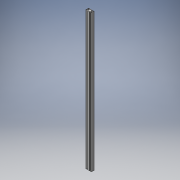
# Autodesk Inventor part: Tslot_2040extrusion_38inch
Saved by Autodesk Inventor 2018 (Build 220112000, 112)
## iProperties
Created: 2020-03-14
Part Number: Tslot_2040extrusion_38inch
Material: Generic
Document SubType Name: Modeling
Designer: natha
Density: 1 g/cm^3
Appearance: Default
Author: natha
Autodesk Inventor part; units mm, degrees
ref_plane "YZ Plane" through (0, 0, 0) normal (1, 0, 0) x (0, 1, 0)
ref_plane "XZ Plane" through (0, 0, 0) normal (0, 1, 0) x (-1, 0, 0)
ref_plane "XY Plane" through (0, 0, 0) normal (0, 0, 1) x (1, 0, 0)
sketch "Sketch1" plane through (0, 0, 0) normal (0, 1, 0) x (-1, 0, 0)
  circle A0 centre (29.9915, -10) radius 2.75
  circle A1 centre (9.9915, -10) radius 2.75
  line L0 (0, 0) -> (0, -6.5)
  line L1 (-0.0085, -20) -> (-0.0085, -13.5)
  line L2 (0, -6.5) -> (0.5, -6.5)
  line L3 (0.5, -6.5) -> (0.5, -7)
  line L4 (0.5, -7) -> (1, -7)
  line L5 (-0.0085, -13.5) -> (0.4915, -13.5)
  line L6 (0.4915, -13.5) -> (0.4915, -13)
  line L7 (0.4915, -13) -> (0.9915, -13)
  line L8 (1, -4.05) -> (3, -4.05)
  line L9 (0.9915, -15.95) -> (2.9915, -15.95)
  line L10 (5.5, -6.5) -> (5.5, -13.5)
  line L11 (5.5, -13.5) -> (2.9915, -15.95)
  line L12 (5.5, -6.5) -> (3, -4.05)
  line L13 (1, -4.05) -> (1, -7)
  line L14 (0.9915, -13) -> (0.9915, -15.95)
  line L15 (-0.0085, -20) -> (6.4915, -20)
  line L16 (6.4915, -20) -> (6.4915, -19.5)
  line L17 (6.4915, -19.5) -> (6.9915, -19.5)
  line L18 (6.9915, -19.5) -> (6.9915, -19)
  line L19 (6.9915, -19) -> (4.0415, -19)
  line L20 (4.0415, -19) -> (4.0415, -17)
  line L21 (13.4915, -20) -> (13.4915, -19.5)
  line L22 (13.4915, -19.5) -> (12.9915, -19.5)
  line L23 (12.9915, -19.5) -> (12.9915, -19)
  line L24 (12.9915, -19) -> (15.9415, -19)
  line L25 (15.9415, -19) -> (15.9415, -17)
  line L26 (15.9415, -17) -> (13.4915, -14.5)
  line L27 (6.4915, -14.5) -> (13.4915, -14.5)
  line L28 (4.0415, -17) -> (6.4915, -14.5)
  line L29 (39.9915, 0) -> (39.9915, -6.5)
  line L30 (39.9915, -6.5) -> (39.4915, -6.5)
  line L31 (39.4915, -6.5) -> (39.4915, -7)
  line L32 (39.4915, -7) -> (38.9915, -7)
  line L33 (38.9915, -7) -> (38.9915, -4.05)
  line L34 (38.9915, -4.05) -> (36.9915, -4.05)
  line L35 (39.9915, -20) -> (39.9915, -13.5)
  line L36 (39.9915, -13.5) -> (39.4915, -13.5)
  line L37 (39.4915, -13.5) -> (39.4915, -13)
  line L38 (39.4915, -13) -> (38.9915, -13)
  line L39 (38.9915, -13) -> (38.9915, -15.95)
  line L40 (38.9915, -15.95) -> (36.9915, -15.95)
  line L41 (34.4915, -6.601) -> (34.4915, -13.5)
  line L42 (34.4915, -13.5) -> (36.9915, -15.95)
  line L43 (34.4915, -6.601) -> (36.9915, -4.05)
  line L44 (39.9915, -20) -> (33.4915, -20)
  line L45 (33.4915, -20) -> (33.4915, -19.5)
  line L46 (33.4915, -19.5) -> (32.9915, -19.5)
  line L47 (32.9915, -19.5) -> (32.9915, -19)
  line L48 (32.9915, -19) -> (35.9415, -19)
  line L49 (35.9415, -19) -> (35.9415, -17)
  line L50 (26.4915, -20) -> (26.4915, -19.5)
  line L51 (26.4915, -19.5) -> (26.9915, -19.5)
  line L52 (26.9915, -19.5) -> (26.9915, -19)
  line L53 (26.9915, -19) -> (24.0415, -19)
  line L54 (24.0415, -19) -> (24.0415, -17)
  line L55 (33.4915, -14.5) -> (26.4915, -14.5)
  line L56 (24.0415, -17) -> (26.4915, -14.5)
  line L57 (33.4915, -14.5) -> (35.9415, -17)
  line L58 (26.4915, -20) -> (13.4915, -20)
  line L59 (39.9915, 0) -> (33.4915, 0)
  line L60 (33.4915, 0) -> (33.4915, -0.5)
  line L61 (33.4915, -0.5) -> (32.9915, -0.5)
  line L62 (32.9915, -0.5) -> (32.9915, -1)
  line L63 (32.9915, -1) -> (35.9415, -1)
  line L64 (35.9415, -1) -> (35.9415, -3)
  line L65 (26.4915, 0) -> (26.4915, -0.5)
  line L66 (26.4915, -0.5) -> (26.9915, -0.5)
  line L67 (26.9915, -0.5) -> (26.9915, -1)
  line L68 (26.9915, -1) -> (24.0415, -1)
  line L69 (24.0415, -1) -> (24.0415, -3)
  line L70 (33.4915, -5.5) -> (26.4915, -5.5)
  line L71 (24.0415, -3) -> (26.4915, -5.5)
  line L72 (35.9415, -3) -> (33.4915, -5.5)
  line L73 (0, 0) -> (6.5, 0)
  line L74 (6.5, 0) -> (6.5, -0.5)
  line L75 (6.5, -0.5) -> (7, -0.5)
  line L76 (7, -0.5) -> (7, -1)
  line L77 (7, -1) -> (4.05, -1)
  line L78 (4.05, -1) -> (4.05, -3)
  line L79 (13.5, 0) -> (13.5, -0.5)
  line L80 (13.5, -0.5) -> (13, -0.5)
  line L81 (13, -0.5) -> (13, -1)
  line L82 (13, -1) -> (15.95, -1)
  line L83 (15.95, -1) -> (15.95, -3)
  line L84 (13.5, -5.5) -> (6.5, -5.5)
  line L85 (6.5, -5.5) -> (4.05, -3)
  line L86 (15.95, -3) -> (13.5, -5.5)
  line L87 (13.5, 0) -> (26.4915, 0)
  dimension "d0" = 40
  dimension "d1" = 20
  dimension "d2" = 5.5
  dimension "d3" = 5.5
  dimension "d4" = 20
  dimension "d11" = 6.5
  dimension "d12" = 6.5
  dimension "d13" = 0.5
  dimension "d14" = 0.5
  dimension "d15" = 0.5
  dimension "d16" = 0.5
  dimension "d17" = 0.5
  dimension "d18" = 0.5
  dimension "d19" = 5.5
  dimension "d20" = 11.9
  dimension "d21" = 6.5
  dimension "d22" = 0.5
  dimension "d23" = 0.5
  dimension "d24" = 0.5
  dimension "d25" = 0.5
  dimension "d26" = 0.5
  dimension "d27" = 0.5
  dimension "d28" = 7
  dimension "d29" = 11.9
  dimension "d31" = 4.05
  dimension "d32" = 2.95
  dimension "d34" = 2
  dimension "d35" = 2
  dimension "d36" = 2
  dimension "d37" = 2
  dimension "d39" = 7
  dimension "d40" = 6.5
  dimension "d41" = 0.5
  dimension "d42" = 0.5
  dimension "d43" = 0.5
  dimension "d44" = 2.95
  dimension "d45" = 2
  dimension "d46" = 6.5
  dimension "d47" = 0.5
  dimension "d48" = 0.5
  dimension "d49" = 0.5
  dimension "d50" = 2.95
  dimension "d51" = 2
  dimension "d52" = 5.5
  dimension "d53" = 6.5
  dimension "d54" = 0.5
  dimension "d55" = 0.5
  dimension "d56" = 0.5
  dimension "d57" = 2.95
  dimension "d58" = 2
  dimension "d59" = 0.5
  dimension "d60" = 0.5
  dimension "d61" = 0.5
  dimension "d62" = 2.95
  dimension "d63" = 2
  dimension "d64" = 7
  dimension "d66" = 6.5
  dimension "d67" = 0.5
  dimension "d68" = 0.5
  dimension "d69" = 0.5
  dimension "d70" = 2.95
  dimension "d71" = 2
  dimension "d72" = 0.5
  dimension "d73" = 0.5
  constraints: 176 end point, 48 perpendicular, 10 horizontal, 9 vertical, 2 centre point, 2 parallel, 1 point on line
  measures "d0" distance of L35.start L1.start
  measures "d1" distance of L29.start L35.start
  measures "d2" diameter of A0
  measures "d3" diameter of A1
  measures "d4" distance of A0.centre A1.centre
  measures "d11" distance of L0.start L0.end
  measures "d12" distance of L1.start L1.end
  measures "d13" distance of L0.end L2.end
  measures "d14" distance of L2.end L3.end
  measures "d15" distance of L3.end L4.end
  measures "d16" distance of L1.end L5.end
  measures "d17" distance of L5.end L6.end
  measures "d18" distance of L6.end L7.end
  measures "d19" distance between parallel lines of L10 L0
  measures "d20" distance between parallel lines of L9 L8
  measures "d21" distance of L1.start L15.end
  measures "d22" distance of L15.end L16.end
  measures "d23" distance of L16.end L17.end
  measures "d24" distance of L17.end L18.end
  measures "d25" distance of L21.start L21.end
  measures "d26" distance of L21.end L22.end
  measures "d27" distance of L22.end L23.end
  measures "d28" distance between parallel lines of L21 L16
  measures "d29" distance between parallel lines of L20 L25
  measures "d31" distance between parallel lines of L20 L1
  measures "d32" distance between parallel lines of L23 L25
  measures "d34" distance of L9.start L9.end
  measures "d35" distance of L8.start L8.end
  measures "d36" distance of L19.end L20.end
  measures "d37" distance of L24.end L25.end
  measures "d39" distance of L27.start L27.end
  measures "d40" distance of L29.start L29.end
  measures "d41" distance of L29.end L30.end
  measures "d42" distance of L30.end L31.end
  measures "d43" distance of L31.end L32.end
  measures "d44" distance of L32.end L33.end
  measures "d45" distance of L33.end L34.end
  measures "d46" distance of L35.start L35.end
  measures "d47" distance of L35.end L36.end
  measures "d48" distance of L36.end L37.end
  measures "d49" distance of L37.end L38.end
  measures "d50" distance of L38.end L39.end
  measures "d51" distance of L39.end L40.end
  measures "d52" distance between parallel lines of L41 L35
  measures "d53" distance of L35.start L44.end
  measures "d54" distance of L44.end L45.end
  measures "d55" distance of L45.end L46.end
  measures "d56" distance of L46.end L47.end
  measures "d57" distance of L47.end L48.end
  measures "d58" distance of L48.end L49.end
  measures "d59" distance of L50.start L50.end
  measures "d60" distance of L50.end L51.end
  measures "d61" distance of L51.end L52.end
  measures "d62" distance of L52.end L53.end
  measures "d63" distance of L53.end L54.end
  measures "d64" distance between parallel lines of L50 L45
  measures "d66" distance of L29.start L59.end
  measures "d67" distance of L59.end L60.end
  measures "d68" distance of L60.end L61.end
  measures "d69" distance of L61.end L62.end
  measures "d70" distance of L62.end L63.end
  measures "d71" distance of L63.end L64.end
  measures "d72" distance of L65.start L65.end
  measures "d73" distance of L65.end L66.end
extrude "Extrusion1" add sketch "Sketch1" along normal blind 965.2
body "Solid1"
